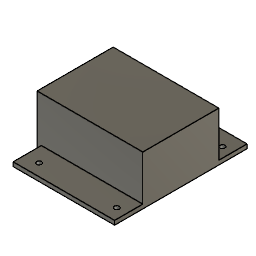
charging_dock_back_2 (Autodesk Fusion 360 design; units mm, degrees)
part number: 2026-07-19-20-43-45-985
Autodesk Fusion 360 part; units mm, degrees
sketch "Sketch1" plane through (0, 0, 0) normal (0, 0, 1) x (1, 0, 0)
  line L0 (70, 0) -> (70, 54)
  line L1 (70, 54) -> (0, 54)
  line L2 (0, 54) -> (0, 0)
  line L3 (5, 49) -> (65, 49)
  line L4 (65, 49) -> (65, 5)
  line L5 (65, 5) -> (5, 5)
  line L6 (5, 5) -> (5, 49)
  line L7 (0, 0) -> (70, 0)
  line L8 (0, 54) -> (70, 54)
  line L9 (70, 54) -> (70, 74)
  line L10 (70, 74) -> (0, 74)
  line L11 (0, 74) -> (0, 54)
  line L12 (0, 0) -> (70, 0)
  line L13 (70, 0) -> (70, -20)
  line L14 (70, -20) -> (0, -20)
  line L15 (0, -20) -> (0, 0)
  dimension "d1" = 54
  dimension "d2" = 70
  dimension "d3" = 5
  dimension "d4" = 5
  dimension "d5" = 5
  dimension "d11" = 5
  dimension "d12" = 20
  dimension "d13" = 20
  constraint vertical L0
  constraint horizontal L1
  constraint vertical L2
  constraint coincident L2.end L7.start
  constraint horizontal L3
  constraint vertical L4
  constraint horizontal L5
  constraint vertical L6
  constraint horizontal L7
  constraint horizontal L8
  constraint vertical L9
  constraint horizontal L10
  constraint vertical L11
  constraint horizontal L12
  constraint vertical L13
  constraint horizontal L14
  constraint vertical L15
  measures "d1" distance of L2.end L1.end
  measures "d2" distance of L2.end L0.start
  measures "d3" distance of L2 L6
  measures "d4" distance of L0 L4
  measures "d5" distance of L1 L3
  measures "d11" distance of L5 L7
  measures "d12" distance of L1.end L10.end
  measures "d13" distance of L2.end L14.end
extrude "Extrude1" add sketch "Sketch1" along normal blind 30 contours L0 L1 L2 L7 L8 L12
extrude "Extrude2" add sketch "Sketch1" along normal blind 3 contours L7 L12 L13 L14 L15 | L1 L8 L9 L10 L11
sketch "Sketch3" plane through (0, 0, 30) normal (0, 0, 1) x (-1, 0, 0)
  line L0 (-65, -5) -> (-5, -5)
  line L1 (-5, -5) -> (-5, -49)
  line L2 (-5, -49) -> (-65, -49)
  line L3 (-65, -49) -> (-65, -5)
  line L4 (0, -54) -> (0, 0)
  line L5 (0, 0) -> (-70, 0)
  line L6 (-70, 0) -> (-70, -54)
  line L7 (-70, -54) -> (0, -54)
  line L8 (0, -54) -> (-70, -54)
  line L9 (-70, -54) -> (-70, 0)
  line L10 (-70, 0) -> (0, 0)
  line L11 (0, 0) -> (0, -54)
  constraint horizontal L8
  constraint vertical L9
  constraint horizontal L10
  constraint vertical L11
  constraint coincident L5.end L6.start
  constraint coincident L4.start L7.end
extrude "Extrude3" add sketch "Sketch3" along normal blind 5 contours L0 L1 L2 L3 | L4 L5 L6 L7 L8 L9 L10 L11
sketch "Sketch4" plane through (0, 0, 3) normal (0, 0, 1) x (-1, 0, 0)
  line L0 (0, -74) -> (0, -54)
  line L1 (0, -54) -> (-70, -54)
  line L2 (-70, -54) -> (-70, -74)
  line L3 (-70, -74) -> (0, -74)
  circle A0 centre (-8, -63.531) radius 1.75
  circle A1 centre (-63, -63.531) radius 1.75
  circle A2 centre (-8, 11.469) radius 1.75
  circle A3 centre (-63, 11.469) radius 1.75
  line L4 (0, -74) -> (0, -54)
  line L5 (-70, -74) -> (0, -74)
  dimension "d18" = 3.5
  dimension "d21" = -55
  dimension "d22" = 75
  dimension "d23" = 8
  dimension "d24" = 10.469
  measures "d18" diameter of A0
  measures "d23" distance of A0.centre L4
  measures "d24" distance of A0.centre L5
extrude "Extrude4" cut sketch "Sketch4" against normal blind 3 contours A0 | A1 | A2 | A3
sketch "Sketch5" plane through (0, 0, 0) normal (-1, 0, 0) x (0, -1, 0)
  line L0 (-74, 0) -> (20, 0)
  line L1 (20, 0) -> (20, 3)
  line L2 (20, 3) -> (0, 3)
  line L3 (0, 3) -> (0, 35)
  line L4 (0, 35) -> (-54, 35)
  line L5 (-54, 35) -> (-54, 3)
  line L6 (-54, 3) -> (-74, 3)
  line L7 (-74, 3) -> (-74, 0)
  line L8 (-5, 0) -> (-49, 0)
  line L9 (-49, 0) -> (-49, 30)
  line L10 (-49, 30) -> (-5, 30)
  line L11 (-5, 30) -> (-5, 0)
  dimension "d27" = 5
  dimension "d28" = 5
  dimension "d33" = 5
  constraint horizontal L8
  constraint vertical L9
  constraint horizontal L10
  constraint vertical L11
  constraint coincident L0 L8.start
  measures "d27" distance of L5 L9
  measures "d28" distance of L3 L11
  measures "d33" distance of L4 L10
extrude "Extrude5" cut sketch "Sketch5" against normal blind 5 contours L0 L8 L9 L10 L11
extrude "Extrude6" add 1 faces at (0, 34.3333, 33.3333) along direction (-1, 0, 0) blind 2
sketch "Sketch7" plane through (-2, 0, 0) normal (-1, 0, 0) x (0, -1, 0)
  line L0 (-5, 30) -> (-5, 0)
  line L1 (-5, 0) -> (20, 0)
  line L2 (20, 0) -> (20, 3)
  line L3 (20, 3) -> (0, 3)
  line L4 (0, 3) -> (0, 35)
  line L5 (0, 35) -> (-54, 35)
  line L6 (-54, 35) -> (-54, 3)
  line L7 (-54, 3) -> (-74, 3)
  line L8 (-74, 3) -> (-74, 0)
  line L9 (-74, 0) -> (-49, 0)
  line L10 (-49, 0) -> (-49, 30)
  line L11 (-49, 30) -> (-5, 30)
  line L12 (-54, 35) -> (0, 35)
  line L13 (0, 35) -> (0, 0)
  line L14 (0, 0) -> (-54, 0)
  line L15 (-54, 0) -> (-54, 35)
  constraint horizontal L12
  constraint vertical L13
  constraint horizontal L14
  constraint vertical L15
  constraint coincident L13.end L14.start
  constraint coincident L5.end L6.start
extrude "Extrude7" add sketch "Sketch7" along normal blind 3 contours L0 L1 L4 L5 L6 L9 L10 L11 L12 L13 L14 L15 | L0 L10 L11 L14
sketch "Sketch8" plane through (-5, 0, 0) normal (-1, 0, 0) x (0, -1, 0)
  line L0 (-54, 0) -> (0, 0)
  line L1 (0, 0) -> (0, 35)
  line L2 (0, 35) -> (-54, 35)
  line L3 (-54, 35) -> (-54, 0)
  line L4 (-36, 0) -> (-20, 0)
  line L5 (-20, 0) -> (-20, 23)
  line L6 (-20, 23) -> (-36, 23)
  line L7 (-36, 23) -> (-36, 0)
  line L8 (-74, 3) -> (-74, 0)
  line L9 (20, 0) -> (20, 3)
  dimension "d39" = 38
  dimension "d40" = 40
  dimension "d41" = 23
  constraint horizontal L4
  constraint vertical L5
  constraint horizontal L6
  constraint vertical L7
  constraint coincident L0 L4.start
  measures "d39" distance of L7 L8
  measures "d40" distance of L5 L9
  measures "d41" distance of L4.end L5.end
extrude "Extrude8" cut sketch "Sketch8" against normal blind 3 contours L0 L4 L5 L6 L7
